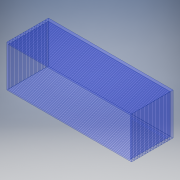
# Autodesk Inventor part: pool cut
Saved by Autodesk Inventor 2019 (Build 230136000, 136)
## iProperties
Created: 2021-05-11
Part Number: pool cut
Material: Steel
Document SubType Name: Modeling
Designer: jamieson-bl
Density: 7.85 g/cm^3
Appearance: Plate
Author: jamieson-bl
Autodesk Inventor part; units mm, degrees
ref_plane "YZ Plane" through (0, 0, 0) normal (1, 0, 0) x (0, 1, 0)
ref_plane "XZ Plane" through (0, 0, 0) normal (0, 1, 0) x (-1, 0, 0)
ref_plane "XY Plane" through (0, 0, 0) normal (0, 0, 1) x (1, 0, 0)
sketch "Sketch1" plane through (0, 0, 0) normal (0, 0, 1) x (1, 0, 0)
  line L0 (2286, -762) -> (-2286, -762)
  line L1 (-2286, -762) -> (-2286, 762)
  line L2 (-2286, 762) -> (2286, 762)
  line L3 (2286, 762) -> (2286, -762)
  line L4 (2286, -762) -> (-2286, 762) construction
  line L5 (-2286, -762) -> (2286, 762) construction
  point P0 (0, 0)
  dimension "d0" = 4572
  dimension "d1" = 1524
  constraints: 12 end point, 2 midpoint, 2 parallel, 1 horizontal, 1 perpendicular
  measures "d0" distance of L1.end L2.end
  measures "d1" distance of L0.end L1.end
extrude "Extrusion1" add sketch "Sketch1" along normal blind 1524
sketch "Sketch2" plane through (0, 0, 1524) normal (0, 0, 1) x (1, 0, 0)
  line L0 (2235.2, -711.2) -> (-2235.2, -711.2)
  line L1 (-2235.2, -711.2) -> (-2235.2, 711.2)
  line L2 (-2235.2, 711.2) -> (2235.2, 711.2)
  line L3 (2235.2, 711.2) -> (2235.2, -711.2)
  line L4 (2235.2, -711.2) -> (-2235.2, 711.2) construction
  line L5 (-2235.2, -711.2) -> (2235.2, 711.2) construction
  point P0 (0, 0)
  dimension "d4" = 4470.4
  dimension "d5" = 1422.4
  constraints: 12 end point, 2 midpoint, 2 parallel, 1 horizontal, 1 perpendicular
  measures "d4" distance of L1.end L2.end
  measures "d5" distance of L0.end L1.end
extrude "Extrusion2" cut sketch "Sketch2" against normal blind 1473.2
sketch "Sketch12" plane through (-2286, 762, 0) normal (0, 1, 0) x (1, 0, 0)
  line L0 (-182.8526, -1524) -> (4734.6574, -1524)
  line L1 (0, -1524) -> (4572, -1524) projected
  line L2 (4734.6574, -1524) -> (4734.6574, -1424)
  line L3 (4734.6574, -1424) -> (-182.8526, -1424)
  line L4 (-182.8526, -1424) -> (-182.8526, -1324)
  line L5 (-182.8526, -1324) -> (4734.6574, -1324)
  line L6 (4734.6574, -1324) -> (4734.6574, -1224)
  line L7 (4734.6574, -1224) -> (-182.8526, -1224)
  line L8 (-182.8526, -1224) -> (-182.8526, -1124)
  line L9 (-182.8526, -1124) -> (4734.6574, -1124)
  line L10 (4734.6574, -1124) -> (4734.6574, -1024)
  line L11 (4734.6574, -1024) -> (-182.8526, -1024)
  line L12 (-182.8526, -1024) -> (-182.8526, -924)
  line L13 (-182.8526, -924) -> (4734.6574, -924)
  line L14 (4734.6574, -924) -> (4734.6574, -824)
  line L15 (4734.6574, -824) -> (-182.8526, -824)
  line L16 (-182.8526, -824) -> (-182.8526, -724)
  line L17 (-182.8526, -724) -> (4734.6574, -724)
  line L18 (4734.6574, -724) -> (4734.6574, -624)
  line L19 (4734.6574, -624) -> (-182.8526, -624)
  line L20 (-182.8526, -624) -> (-182.8526, -524)
  line L21 (-182.8526, -524) -> (4734.6574, -524)
  line L22 (4734.6574, -524) -> (4734.6574, -424)
  line L23 (4734.6574, -424) -> (-182.8526, -424)
  line L24 (-182.8526, -424) -> (-182.8526, -324)
  line L25 (-182.8526, -324) -> (4734.6574, -324)
  line L26 (4734.6574, -324) -> (4734.6574, -224)
  line L27 (4734.6574, -224) -> (-182.8526, -224)
  line L28 (-182.8526, -224) -> (-182.8526, -124)
  line L29 (-182.8526, -124) -> (4734.6574, -124)
  point P0 (2286, 0)
  dimension "d46" = 100
  dimension "d47" = 100
  dimension "d48" = 100
  dimension "d49" = 100
  dimension "d50" = 100
  dimension "d51" = 100
  dimension "d52" = 100
  dimension "d53" = 100
  dimension "d54" = 100
  dimension "d55" = 100
  dimension "d56" = 100
  dimension "d57" = 100
  dimension "d58" = 100
  dimension "d59" = 100
  constraints: 58 end point, 25 point on line, 11 perpendicular, 5 parallel, 1 collinear
  measures "d46" distance of L0.end L2.end
  measures "d47" distance of L3.end L4.end
  measures "d48" distance of L5.end L6.end
  measures "d49" distance of L7.end L8.end
  measures "d50" distance of L9.end L10.end
  measures "d51" distance of L11.end L12.end
  measures "d52" distance of L13.end L14.end
  measures "d53" distance of L15.end L16.end
  measures "d54" distance of L17.end L18.end
  measures "d55" distance of L19.end L20.end
  measures "d56" distance of L21.end L22.end
  measures "d57" distance of L23.end L24.end
  measures "d58" distance of L25.end L26.end
  measures "d59" distance of L27.end L28.end
split_face "Split8"
body "Solid1"
